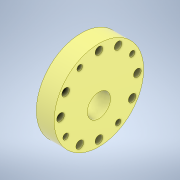
# Autodesk Inventor part: sample-transfer_insulation
Saved by Autodesk Inventor 2020 (Build 240168000, 168)
## iProperties
Created: 2019-08-16
Part Number: sample-transfer_insulation
Material: ABS Plastic light yellow
Document SubType Name: Modeling
Designer: rainer
Density: 1.06 g/cm^3
Appearance: Smooth - White(1)
Author: rainer
Autodesk Inventor part; units mm, degrees
ref_plane "YZ Plane" through (0, 0, 0) normal (1, 0, 0) x (0, 1, 0)
ref_plane "XZ Plane" through (0, 0, 0) normal (0, 1, 0) x (-1, 0, 0)
ref_plane "XY Plane" through (0, 0, 0) normal (0, 0, 1) x (1, 0, 0)
sketch "Sketch1" plane through (0, 0, 0) normal (1, 0, 0) x (0, 1, 0)
  circle A0 centre (0, 0) radius 34.95
  circle A1 centre (-6.9, 0) radius 9.05
  dimension "d0" = 69.9
  dimension "d1" = 18.1
  dimension "d2" = 6.9
  constraints: 2 centre point, 1 coincident
  measures "d0" diameter of A0
  measures "d1" diameter of A1
  measures "d2" distance of point (0, 0) A1.centre
extrude "Extrusion1" add sketch "Sketch1" along normal blind 13.9
sketch "Sketch2" plane through (13.9, 0, 0) normal (1, 0, 0) x (0, 0, -1)
  circle A0 centre (0, 0) radius 30
  point P0 (0, 30)
  dimension "d5" = 60
  constraints: 1 coincident, 1 vertical alignment, 2 other
hole "Hole1" at (13.9, 30, 0) direction (-1, 0, 0) diameter 4.4 depth 13.9 counterbore diameter 6 counterbore depth 8.9
pattern_circular "Circular Pattern1" count 4 over 360 about axis through (0, 0, 0) along (1, 0, 0) of "Hole1"
sketch "Sketch4" plane through (0, 0, 0) normal (-1, 0, 0) x (0, 0, 1)
  circle A0 centre (0, 0) radius 30
  line L0 (0, 0) -> (25.9808, 15)
  line L1 (0, 0) -> (30, 0) construction
  dimension "d28" = 60
  dimension "d29" = 30
  constraints: 4 end point, 2 coincident, 1 equal length, 1 horizontal, 3 other
  measures "d29" angle of L1 L0
hole "Hole3" at (0, 15, 25.9808) direction (1, 0, 0) diameter 6 end through all
pattern_circular "Circular Pattern3" count 4 over 360 about axis through (0, 0, 0) along (1, 0, 0) of "Hole3"
sketch "Sketch5" plane through (0, 0, 0) normal (-1, 0, 0) x (0, 0, 1)
  circle A0 centre (0, 0) radius 30
  line L0 (0, 0) -> (15, 25.9808)
  line L1 (0, 0) -> (30, 0) construction
  point P0 (15, 25.9808)
  dimension "d40" = 60
  dimension "d41" = 60
  constraints: 4 end point, 2 point on circle, 1 centre point, 1 coincident, 1 equal length, 1 horizontal
  measures "d40" diameter of A0
  measures "d41" angle of L1 L0
hole "Hole4" at (0, 25.9808, 15) direction (1, 0, 0) diameter 4.4 depth 13.9 counterbore diameter 6 counterbore depth 8.9
pattern_circular "Circular Pattern4" count 4 over 360 about axis through (0, 0, 0) along (1, 0, 0) of "Hole4"
body "Solid1"
